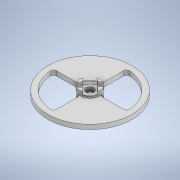
# Autodesk Inventor part: Lucka Överdel
Saved by Autodesk Inventor 2021 (Build 250183000, 183)
## iProperties
Created: 2025-01-13
Part Number: Lucka Överdel
Material: Generic
Document SubType Name: Sheet Metal
Designer: 24oscnor
Density: 1 g/cm^3
Sheet Metal Rule: Default_mm
Appearance: Default
Author: 24oscnor
## iProperties of the stored document _3DPrint.ipt
Created: 2025-01-15
Part Number: _3DPrint
Material: Generic
Document SubType Name: Modeling
Designer: 24oscnor
Density: 1 g/cm^3
Appearance: Default
Author: 24oscnor
Autodesk Inventor part; units mm, degrees
ref_plane "YZ Plane" through (0, 0, 0) normal (1, 0, 0) x (0, 1, 0)
ref_plane "XZ Plane" through (0, 0, 0) normal (0, 1, 0) x (-1, 0, 0)
ref_plane "XY Plane" through (0, 0, 0) normal (0, 0, 1) x (1, 0, 0)
sketch "Sketch1" plane through (0, 0, 0) normal (0, 1, 0) x (-1, 0, 0)
  circle A0 centre (0, 0) radius 27.5
  line L0 (0, 0) -> (0, 27.5)
  line L1 (0, 0) -> (0, -27.5)
  line L2 (0, 0) -> (-27.5, 0)
  line L3 (0, 0) -> (27.5, 0)
  circle A1 centre (0, 0) radius 24
  circle A2 centre (0, 0) radius 2.55
  circle A3 centre (0, 0) radius 6.5
  point P0 (24, 0)
  point P1 (2.55, 0)
  point P2 (0, -2.55)
  point P3 (0, -24)
  point P4 (-24, 0)
  point P5 (-2.55, 0)
  point P6 (0, 2.55)
  point P7 (0, 24)
  point P8 (-6.5, 0)
  point P9 (0, -6.5)
  point P10 (6.5, 0)
  point P11 (0, 6.5)
  dimension "d0" = 55
  dimension "d1" = 48
  dimension "d2" = 5.1
  dimension "d5" = 13
  constraints: 8 end point, 4 centre point, 4 coincident, 4 point on circle, 2 point on line, 1 perpendicular, 1 vertical
  measures "d0" diameter of A0
  measures "d1" diameter of A1
  measures "d2" diameter of A2
  measures "d5" diameter of A3
extrude "Extrusion1" add sketch "Sketch1" along normal blind 3 contours L3 A1 L0 A0 | A0 L1 A1 L3 | L0 A1 L2 A0 | A0 L2 A1 L1 | A1 L1 A3 L3 | L0 A3 L2 A1 | A3 L1 A2 L3 | L3 A2 L0 A3 | L0 A2 L2 A3 | A3 L2 A2 L1
fillet "Fillet1" radius 2 8 edges at (-6.5, 1.5, 0) (0, 1.5, 6.5) (-24, 1.5, 0) (0, 1.5, 24) (0, 1.5, -24) (0, 1.5, -6.5) (24, 1.5, 0) (6.5, 1.5, 0)
sketch "Sketch2" plane through (0, 3, 0) normal (0, 1, 0) x (1, 0, 0)
  circle A0 centre (0, 0) radius 6.5
  dimension "d7" = 13
  constraints: 1 centre point, 1 coincident
  measures "d7" diameter of A0
extrude "Extrusion2" add sketch "Sketch2" along normal blind 3
sketch "Sketch3" plane through (0, 6, 0) normal (0, 1, 0) x (1, 0, 0)
  point P0 (0, 0)
sketch "Sketch4" plane through (0, 6, 0) normal (0, 1, 0) x (1, 0, 0)
  circle A0 centre (0, 0) radius 6.5 projected
  line L0 (5.6288, 3.2506) -> (-2.6597, -5.9309)
  line L1 (-5.6288, -3.2506) -> (2.6597, 5.9309)
  arc A1 (-1.5294, -6.3175) -> (6.3175, 1.5294) centre (0, 0) ccw projected
  line L2 (6.384, -1.2224) -> (-1.5727, 6.3069)
  arc A2 (1.5294, 6.3175) -> (-6.3175, -1.5294) centre (0, 0) ccw projected
  line L3 (-6.384, 1.2224) -> (1.5727, -6.3069)
  point P0 (-3.799, -1.2237)
  point P1 (-0.8928, -3.9737)
  point P2 (3.799, 1.2237)
  point P3 (0.8928, 3.9737)
  point P4 (-1.5727, 6.3069)
  dimension "d10" = 4
  dimension "d11" = 2
  dimension "d12" = 7
  dimension "d13" = 3.5
  constraints: 8 end point, 2 point on circle, 1 parallel, 7 other
  measures "d10" distance between parallel lines of L0 L1
  measures "d11" distance from line of point (0, 0) L1
  measures "d12" distance between parallel lines of L2 L3
  measures "d13" distance from line of point (0, 0) L3
extrude "Extrusion3" cut sketch "Sketch4" against normal blind 2 contours A0 L3 L0 L2 | L0 L2 L1 A0 | L0 L3 L1 L2 | L0 A0 L1 L3 | L1 L3 A0 L2
sketch "Sketch5" plane through (0, 4, 0) normal (0, 1, 0) x (1, 0, 0)
  arc A0 (1.5727, -6.3069) -> (6.384, -1.2224) centre (0, 0) ccw projected
  line L0 (-3.799, -1.2237) -> (-6.384, 1.2224) projected
  line L1 (1.5727, -6.3069) -> (-6.384, 1.2224)
  arc A1 (-1.5727, 6.3069) -> (-6.384, 1.2224) centre (0, 0) ccw projected
  line L2 (-6.384, 1.2224) -> (-1.5727, 6.3069)
  line L3 (-1.5727, 6.3069) -> (6.384, -1.2224)
  line L4 (6.384, -1.2224) -> (1.5727, -6.3069)
  constraints: 8 end point, 3 perpendicular, 1 collinear
extrude "Extrusion4" cut sketch "Sketch5" against normal blind 1 contours L1 L0 L2 L3 L4
sketch "Sketch7" plane through (-3.799, 4, 1.2237) normal (0.6873266, 0, -0.7263485) x (-0.7263485, 0, -0.6873266)
  line L0 (3.5589, -1) -> (3.5589, 0) projected
  line L1 (-7.3956, -1) -> (3.5589, -1) projected
  line L2 (3.5589, 0) -> (2.3243, -1)
  line L3 (-3.671, -1) -> (3.5589, -1) projected
  line L4 (2.3243, -1) -> (3.5589, -1)
  line L5 (3.5589, -1) -> (3.5589, 0)
  line L6 (-7.3956, 0) -> (-7.3956, 2) projected
  line L7 (-7.3956, -1) -> (3.5589, -1) projected
  line L8 (-7.3956, 0) -> (-6.161, -1)
  line L9 (-7.3956, -1) -> (-5.1497, -1) projected
  line L10 (-6.161, -1) -> (-7.3956, -1)
  line L11 (-7.3956, -1) -> (-7.3956, 0)
  point P0 (-1.9184, -4)
  constraints: 12 end point, 2 collinear, 2 perpendicular, 2 point on line
extrude "Extrusion5" add sketch "Sketch7" along normal up to next
equation "\"BendRadius\" = Thickness"
equation "\"BendReliefWidth\" = Thickness"
equation "\"BendReliefDepth\" = 0.5 * Thickness"
equation "\"CornerReliefSize\" = 4 * Thickness"
equation "\"MinimumRemnant\" = 2 * Thickness"
equation "\"TransitionRadius\" = BendRadius"
equation "\"JacobiRadiusSize\" = BendRadius"
equation "\"GapSize\" = Thickness"
equation "\"Thickness\" = 0.5"
body "Solid1"
